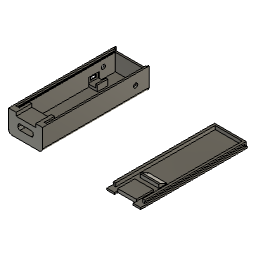
Coco_long_flat_Cover (Autodesk Fusion 360 design; units mm, degrees)
Autodesk Fusion 360 part; units mm, degrees
sketch "Skizze1" plane through (0, 0, 0) normal (0, 0, 1) x (1, 0, 0)
  line L0 (18, 20) -> (38, 20)
  line L1 (38, 20) -> (38, 83)
  line L2 (38, 83) -> (18, 83)
  line L3 (18, 83) -> (18, 20)
  line L4 (19, 23.2) -> (37, 23.2)
  line L5 (37, 23.2) -> (37, 82)
  line L6 (37, 82) -> (19, 82)
  line L7 (19, 82) -> (19, 23.2)
  line L8 (57, 90.4333) -> (57, 15.7858)
  line L9 (77, 82) -> (95, 82)
  line L10 (76, 83) -> (96, 83)
  line L11 (96, 83) -> (96, 20)
  line L12 (77, 23.2) -> (77, 82)
  line L13 (96, 20) -> (76, 20)
  line L14 (95, 82) -> (95, 23.2)
  line L15 (76, 20) -> (76, 83)
  line L16 (78, 81) -> (94, 81)
  line L17 (94, 81) -> (94, 23.2)
  line L18 (78, 23.2) -> (78, 81)
  line L19 (78, 81) -> (78, 83)
  line L20 (94, 81) -> (94, 83)
  line L21 (95, 82) -> (95, 83)
  line L22 (77, 82) -> (77, 83)
  line L23 (95, 23.2) -> (94, 23.2)
  line L24 (77, 23.2) -> (78, 23.2)
  line L25 (-15, -7.8) -> (-15, -6.8)
  line L26 (-15, -6.8) -> (-13, -6.8)
  line L27 (-13, -6.8) -> (-13, -15)
  line L28 (-13, -15) -> (-15, -15)
  line L29 (-15, -15) -> (-15, -14)
  line L30 (-15, -14) -> (-13.6, -14)
  line L31 (-13.6, -14) -> (-13.6, -7.8)
  line L32 (-13.6, -7.8) -> (-15, -7.8)
  dimension "d3" = 63
  dimension "d4" = 20
  dimension "d5" = 1
  dimension "d6" = 1
  dimension "d7" = 19
  dimension "d8" = 59.8
  dimension "d13" = 1
  dimension "d15" = 1
  dimension "d16" = 17
  dimension "d71" = 38
  dimension "d72" = 83
  dimension "d212" = 15
  dimension "d213" = 15
  dimension "d214" = 1
  dimension "d215" = 2
  dimension "d216" = 1.4
  dimension "d217" = 7.2
  dimension "d218" = 8.2
  dimension "d246" = 114
  constraint horizontal L0
  constraint vertical L1
  constraint horizontal L2
  constraint vertical L3
  constraint horizontal L4
  constraint vertical L5
  constraint horizontal L6
  constraint vertical L7
  constraint vertical L8
  constraint symmetric L0.start L8 L11.end
  constraint symmetric L0.end L8 L13.end
  constraint symmetric L1.end L8 L10.start
  constraint symmetric L2.end L8 L10.end
  constraint symmetric L4.start L8 L14.end
  constraint symmetric L4.end L8 L12.start
  constraint symmetric L5.end L8 L9.start
  constraint symmetric L6.end L8 L9.end
  constraint horizontal L16
  constraint vertical L17
  constraint vertical L18
  constraint coincident L10 L19.end
  constraint perpendicular L10 L19
  constraint coincident L10 L20.end
  constraint perpendicular L10 L20
  constraint coincident L10 L21.end
  constraint perpendicular L10 L21
  constraint coincident L10 L22.end
  constraint perpendicular L10 L22
  constraint perpendicular L14 L23
  constraint perpendicular L12 L24
  constraint vertical L25
  constraint perpendicular L25 L26
  constraint perpendicular L26 L27
  constraint perpendicular L27 L28
  constraint perpendicular L28 L29
  constraint perpendicular L27 L30
  constraint perpendicular L30 L31
  constraint perpendicular L25 L32
  constraint collinear L25 L29
  measures "d3" distance of L0 L2
  measures "d4" distance of L1 L3
  measures "d5" distance of L2 L6
  measures "d6" distance of L1 L5
  measures "d7" distance of L1 L7
  measures "d8" distance of L2 L4
  measures "d13" distance of L9 L16
  measures "d15" distance of L14 L17
  measures "d16" distance of L14 L18
  measures "d71" distance of origin L1
  measures "d72" distance of origin L2
  measures "d212" distance of origin L28
  measures "d213" distance of origin L29
  measures "d214" distance of L28 L30
  measures "d215" distance of L27 L29
  measures "d216" distance of L29 L31
  measures "d217" distance of L28 L32
  measures "d218" distance of L26 L28
extrude "Extrusion1" add sketch "Skizze1" along normal blind 13 contours L0 L1 L2 L3 makes body 1
extrude "Extrusion2" add sketch "Skizze1" along normal blind 1 contours L4 L5 L6 L7 bodies 1
extrude "Extrusion3" add sketch "Skizze1" along normal blind 3 separate body contours L9 L10 L19 L22 | L9 L12 L18 L19 L24 | L9 L10 L19 L20 | L9 L10 L20 L21 | L9 L14 L17 L20 L23 makes body 2
extrude "Extrusion4" add sketch "Skizze1" along normal blind 1 contours L9 L10 L19 L22 | L10 L11 L12 L13 L14 L15 L16 L17 L18 L21 L22 L23 L24 | L9 L10 L19 L20 | L9 L16 L19 L20 | L9 L10 L20 L21 bodies 2
fillet "Abrundung1" radius 2 2 edges at (38, 51.5, 0) (18, 51.5, 0) on bodies 1
ref_plane "Arbeitsebene1" through (28, 0, 0) normal (1, 0, 0) x (0, 1, 0)
sketch "Skizze2" plane through (28, 0, 0) normal (1, 0, 0) x (0, 1, 0)
  line L0 (23.2, 12) -> (83, 12)
  line L1 (83, 12) -> (83, 11)
  line L2 (83, 11) -> (23.2, 11)
  line L3 (23.2, 11) -> (23.2, 12)
  dimension "d25" = 11
  dimension "d26" = 59.8
  dimension "d27" = 1
  dimension "d44" = 83
  constraint horizontal L0
  constraint vertical L1
  constraint horizontal L2
  constraint vertical L3
  measures "d25" vertical distance of origin L2.end
  measures "d26" distance of L1 L3
  measures "d27" distance of L0 L2
  measures "d44" distance of origin L1
extrude "Extrusion10" cut sketch "Skizze2" along normal mid plane 19 bodies 1
sketch "Skizze3" plane through (0, 20, 0) normal (0, -1, 0) x (1, 0, 0)
  arc A0 (18, 2) -> (20, 0) centre (20, 2) ccw
  line L0 (20, 0) -> (36, 0)
  arc A1 (36, 0) -> (38, 2) centre (36, 2) ccw
  line L1 (38, 2) -> (38, 13)
  line L2 (38, 13) -> (18, 13)
  line L3 (18, 13) -> (18, 2)
  line L4 (24.69, 4.89) -> (31.31, 4.89)
  line L5 (24.69, 8.11) -> (31.31, 8.11)
  line L6 (28, 12.5188) -> (28, 0.4317)
  arc A2 (23.49, 6.09) -> (24.69, 4.89) centre (24.69, 6.09) ccw
  line L7 (23.49, 6.09) -> (23.49, 6.91)
  arc A3 (24.69, 8.11) -> (23.49, 6.91) centre (24.69, 6.91) ccw
  arc A4 (32.51, 6.91) -> (31.31, 8.11) centre (31.31, 6.91) ccw
  arc A5 (31.31, 4.89) -> (32.51, 6.09) centre (31.31, 6.09) ccw
  line L8 (32.51, 6.91) -> (32.51, 6.09)
  line L9 (22.5, 13) -> (34, 13)
  line L10 (34, 13) -> (34, 11)
  line L11 (34, 11) -> (22.5, 11)
  line L12 (22.5, 11) -> (22.5, 13)
  dimension "d30" = 6.62
  dimension "d31" = 4.89
  dimension "d32" = 6.62
  dimension "d33" = 8.11
  dimension "d34" = 3.31
  dimension "d35" = 3.31
  dimension "d36" = 1.2
  dimension "d37" = 1.2
  dimension "d171" = 2
  dimension "d204" = 6
  dimension "d205" = 11.5
  constraint horizontal L4
  constraint horizontal L5
  constraint tangent L4 A2
  constraint vertical L7
  constraint tangent L7 A3
  constraint tangent L5 A3
  constraint tangent A2 L7
  constraint tangent L5 A4
  constraint tangent L4 A5
  constraint perpendicular L2 L8
  constraint tangent A5 L8
  constraint tangent A4 L8
  constraint horizontal L9
  constraint vertical L10
  constraint horizontal L11
  constraint vertical L12
  constraint coincident L2 L9.start
  measures "d30" distance of L4.start L4.end
  measures "d31" distance of L0 L4
  measures "d32" distance of L5.start L5.end
  measures "d33" distance of L0 L5
  measures "d34" distance of L4.end L6
  measures "d35" distance of L5.end L6
  measures "d36" radius of A3
  measures "d37" radius of A4
  measures "d171" distance of L9 L11
  measures "d204" distance of L6 L10
  measures "d205" distance of L10 L12
extrude "Extrusion6" cut sketch "Skizze3" against normal blind 3.2 contours L2 L9 L10 L11 L12 | L4 L5 L6 A2 L7 A3 | L4 L5 L6 A4 A5 L8 bodies 1
fillet "Abrundung2" [suppressed]
sketch "Skizze7" plane through (0, 83, 0) normal (0, 1, 0) x (-1, 0, 0)
  arc A0 (-20, 0) -> (-18, 2) centre (-20, 2) ccw
  line L0 (-18, 2) -> (-18, 13)
  line L1 (-38, 13) -> (-38, 2)
  arc A1 (-38, 2) -> (-36, 0) centre (-36, 2) ccw
  line L2 (-36, 0) -> (-20, 0)
  line L3 (-37.5, 13) -> (-18.5, 13)
  line L4 (-18.5, 13) -> (-18.5, 12)
  line L5 (-18.5, 12) -> (-37.5, 12)
  line L6 (-37.5, 12) -> (-37.5, 13)
  line L7 (-28, 12.5188) -> (-28, 0.4317)
  circle A2 centre (-31.5, 6) radius 1.25
  line L8 (-18.5, 11) -> (-37.5, 11)
  line L9 (-18.5, 12) -> (-18.5, 11)
  line L10 (-37.5, 11) -> (-37.5, 12)
  line L11 (-37.5, 12) -> (-18.5, 12)
  line L12 (-18, 13) -> (-38, 13)
  dimension "d59" = 19
  dimension "d60" = 9.5
  dimension "d116" = 2.5
  dimension "d117" = 6
  dimension "d206" = 3.5
  dimension "d264" = 13
  dimension "d265" = 1
  constraint horizontal L3
  constraint vertical L4
  constraint horizontal L5
  constraint vertical L6
  measures "d59" distance of L4 L6
  measures "d60" distance of L4 L7
  measures "d116" diameter of A2
  measures "d117" distance of L2 A2.centre
  measures "d206" distance of L7 A2.centre
  measures "d264" distance of origin L3
  measures "d265" distance of L3 L5
extrude "Extrusion11" cut sketch "Skizze7" against normal blind 1 contours L3 L4 L5 L6 L11 L12 bodies 1
sketch "Skizze8" plane through (95, 0, 0) normal (1, 0, 0) x (0, 1, 0)
  line L0 (23.2, 1) -> (83, 1)
  line L1 (83, 1) -> (83, 3)
  line L2 (83, 3) -> (23.2, 3)
  line L3 (23.2, 3) -> (83, 3)
  line L4 (82, 2.1) -> (23.2, 2.1)
  line L5 (23.2, 2.1) -> (23.2, 3)
  line L6 (83, 3) -> (83, 1)
  line L7 (82, 1) -> (82, 2.1)
  line L8 (23.2, 3) -> (23.2, 1)
  dimension "d63" = 0.9
  dimension "d125" = 1
  constraint horizontal L3
  constraint horizontal L4
  constraint vertical L5
  constraint coincident L2.end L3.start
  constraint coincident L0.end L1.start
  constraint coincident L0 L7.start
  constraint coincident L4 L7.end
  constraint perpendicular L4 L7
  constraint coincident L1.end L2.start
  measures "d63" distance of L2.end L4.end
  measures "d125" distance of L6 L7
extrude "Extrusion12" add sketch "Skizze8" along normal blind 0.4 contours L0 L1 L2 L3 L4 L5 L6 L7 L8 bodies 2
sketch "Skizze9" plane through (77, 0, 0) normal (-1, 0, 0) x (0, -1, 0)
  line L0 (-83, 1) -> (-23.2, 1)
  line L1 (-23.2, 3) -> (-83, 3)
  line L2 (-83, 3) -> (-83, 1)
  line L3 (-83, 3) -> (-23.2, 3)
  line L4 (-23.2, 3) -> (-23.2, 2.1)
  line L5 (-23.2, 2.1) -> (-82, 2.1)
  line L6 (-83, 1) -> (-83, 3)
  line L7 (-83, 1) -> (-82, 1)
  line L8 (-82, 2.1) -> (-82, 1)
  line L9 (-23.2, 1) -> (-23.2, 3)
  line L10 (-83, 1) -> (-23.2, 1)
  line L11 (-23.2, 1) -> (-23.2, 3)
  line L12 (-23.2, 3) -> (-83, 3)
  line L13 (-83, 3) -> (-83, 1)
  dimension "d126" = 0.9
  dimension "d127" = 1
  constraint horizontal L3
  constraint vertical L4
  constraint horizontal L5
  constraint vertical L6
  constraint coincident L1.end L2.start
  constraint coincident L0.start L2.end
  constraint coincident L0 L7.end
  constraint coincident L5 L8.start
  constraint perpendicular L0 L8
  constraint coincident L5.end L8
  constraint coincident L1.start L3.end
  measures "d126" distance of L3 L5
  measures "d127" distance of L6 L8
extrude "Extrusion13" add sketch "Skizze9" along normal blind 0.4 contours L0 L1 L2 L3 L4 L5 L6 L7 L8 L9 L10 L11 L12 L13 bodies 2
sketch "Skizze10" plane through (0, 0, 1) normal (0, 0, 1) x (-1, 0, 0)
  line L0 (-76.6, -83) -> (-76, -83)
  line L1 (-76, -20) -> (-96, -20)
  line L2 (-95, -82) -> (-95, -23.2)
  line L3 (-94, -23.2) -> (-94, -82)
  line L4 (-95, -23.2) -> (-94, -23.2)
  line L5 (-95.4, -82) -> (-95, -82)
  line L6 (-95.4, -83) -> (-95.4, -82)
  line L7 (-76, -83) -> (-76, -20)
  line L8 (-96, -20) -> (-96, -83)
  line L9 (-96, -83) -> (-95.4, -83)
  line L10 (-80.5, -32) -> (-91.5, -32)
  line L11 (-80.5, -32) -> (-80.5, -22)
  line L12 (-80.5, -22) -> (-91.5, -22)
  line L13 (-91.5, -22) -> (-91.5, -32)
  line L14 (-80.5, -40.2) -> (-91.5, -40.2)
  line L15 (-91.5, -40.2) -> (-91.5, -35.2)
  line L16 (-91.5, -35.2) -> (-80.5, -35.2)
  line L17 (-80.5, -35.2) -> (-80.5, -40.2)
  line L18 (-77, -23.2) -> (-77, -82)
  line L19 (-78, -82) -> (-78, -23.2)
  line L20 (-78, -23.2) -> (-77, -23.2)
  line L21 (-76.6, -83) -> (-95.4, -83)
  line L22 (-76.6, -82) -> (-76.6, -83)
  line L23 (-77, -82) -> (-76.6, -82)
  dimension "d224" = 4.5
  dimension "d225" = 15.5
  dimension "d226" = 2
  dimension "d227" = 12
  dimension "d249" = 20.2
  dimension "d250" = 15.2
  constraint perpendicular L10 L11
  constraint perpendicular L10 L13
  constraint horizontal L14
  constraint vertical L15
  constraint horizontal L16
  constraint vertical L17
  constraint collinear L11 L17
  constraint collinear L13 L15
  measures "d224" distance of L7 L11
  measures "d225" distance of L7 L13
  measures "d226" distance of L1 L12
  measures "d227" distance of L1 L10
  measures "d249" distance of L1 L14
  measures "d250" distance of L1 L16
extrude "Extrusion30" add sketch "Skizze10" along normal blind 1 contours L10 L11 L12 L13 bodies 2
extrude "Extrusion33" add sketch "Skizze10" along normal blind 2 contours L14 L15 L16 L17 bodies 2
chamfer "Fase2" distance 4 distance2 2 1 edges at (86, 40.2, 3) measured on face at (84.1667, 38.5333, 3) on bodies 2
sketch "Skizze11" plane through (18, 0, 0) normal (-1, 0, 0) x (0, -1, 0)
  line L0 (-83, 2) -> (-20, 2)
  line L1 (-20, 2) -> (-20, 13)
  line L2 (-20, 13) -> (-83, 13)
  line L3 (-83, 13) -> (-83, 2)
  line L4 (-71.2, 3.4) -> (-67.9, 3.4)
  line L5 (-67.9, 3.4) -> (-67.9, 5)
  line L6 (-67.9, 5) -> (-71.2, 5)
  line L7 (-71.2, 5) -> (-71.2, 3.4)
  line L8 (-66.5, 5.95) -> (-66.5, 2.45)
  line L9 (-66.5, 5.95) -> (-72.6, 5.95)
  line L10 (-72.6, 5.95) -> (-72.6, 2.45)
  line L11 (-72.6, 2.45) -> (-66.5, 2.45)
  circle A0 centre (-75, 7) radius 1.25
  dimension "d76" = 3.3
  dimension "d77" = 1.6
  dimension "d78" = 15.1
  dimension "d179" = 3.95
  dimension "d180" = 3.5
  dimension "d181" = 16.5
  dimension "d182" = 6.1
  dimension "d193" = 3
  dimension "d258" = 6
  dimension "d259" = 8
  dimension "d260" = 2.5
  constraint horizontal L4
  constraint vertical L5
  constraint horizontal L6
  constraint vertical L7
  constraint perpendicular L6 L8
  constraint perpendicular L8 L9
  constraint perpendicular L0 L10
  constraint horizontal L11
  measures "d76" distance of L4.start L4.end
  measures "d77" distance of L4.start L6.end
  measures "d78" distance of L3 L5
  measures "d179" distance of L0 L9
  measures "d180" distance of L9 L11
  measures "d181" distance of L3 L8
  measures "d182" distance of L8 L10
  measures "d193" distance of L0 L6
  measures "d258" distance of L2 A0.centre
  measures "d259" distance of L3 A0.centre
  measures "d260" diameter of A0
extrude "Extrusion15" cut sketch "Skizze11" against normal blind 1 contours L4 L5 L6 L7 bodies 1
extrude "Extrusion34" cut sketch "Skizze11" against normal blind 20 contours A0 bodies 1
sketch "Skizze12" plane through (0, 0, 1) normal (0, 0, 1) x (-1, 0, 0)
  line L0 (-19, -82) -> (-19, -23.2)
  line L1 (-19, -23.2) -> (-37, -23.2)
  line L2 (-37, -23.2) -> (-37, -82)
  line L3 (-23, -72.5) -> (-23, -66.4)
  line L4 (-24, -72.5) -> (-24, -66.4)
  line L5 (-24, -66.4) -> (-23, -66.4)
  line L6 (-34, -20) -> (-38, -20)
  line L7 (-18, -20) -> (-22.5, -20)
  line L8 (-24, -72.5) -> (-23, -72.5)
  line L9 (-18, -83) -> (-18, -20)
  line L10 (-23, -72.5) -> (-19, -72.5)
  line L11 (-23, -66.4) -> (-19, -66.4)
  line L12 (-18.5, -83) -> (-18, -83)
  dimension "d177" = 6
  dimension "d178" = 5
  dimension "d253" = 10.5
  dimension "d254" = 16.6
  constraint vertical L3
  constraint perpendicular L4 L5
  constraint vertical L4
  constraint perpendicular L3 L8
  constraint coincident L0 L10.end
  constraint perpendicular L0 L10
  constraint coincident L0 L11.end
  constraint perpendicular L0 L11
  measures "d177" distance of L4 L9
  measures "d178" distance of L3 L9
  measures "d253" distance of L10 L12
  measures "d254" distance of L11 L12
extrude "Extrusion17" add sketch "Skizze12" along normal blind 3.5 contours L3 L4 L5 L8 bodies 1
extrude "Extrusion27" add sketch "Skizze12" along normal blind 1.45 contours L0 L3 L10 L11 bodies 1
sketch "Skizze13" plane through (19, 0, 0) normal (1, 0, 0) x (0, 1, 0)
  line L0 (82, 1) -> (82, 11)
  line L1 (23.2, 11) -> (23.2, 1)
  line L2 (72.5, 1) -> (82, 1)
  line L3 (71.2, 3.4) -> (67.9, 3.4)
  line L4 (67.9, 3.4) -> (67.9, 5)
  line L5 (67.9, 5) -> (71.2, 5)
  line L6 (71.2, 5) -> (71.2, 3.4)
  line L7 (-70.5, 1.05) -> (-64.4, 1.05)
  line L8 (-64.4, 4.55) -> (-64.4, 1.05)
  line L9 (-65.9, 2) -> (-65.9, 3.6)
  line L10 (-69, 2) -> (-65.9, 2)
  line L11 (-64.4, 4.55) -> (-70.5, 4.55)
  line L12 (-70.5, 4.55) -> (-70.5, 1.05)
  line L13 (-69, 3.6) -> (-69, 2)
  line L14 (-65.9, 3.6) -> (-69, 3.6)
  line L15 (66.4, 5.95) -> (66.4, 1)
  line L16 (72.5, 1) -> (72.5, 5.95)
  line L17 (72.5, 5.95) -> (66.4, 5.95)
  line L18 (83, 13) -> (83, 2)
  line L19 (72.6, 2.45) -> (66.5, 2.45)
  line L20 (72.5, 2.45) -> (72.5, 1)
  line L21 (66.4, 1) -> (66.4, 2.45)
  line L22 (66.4, 2.45) -> (72.5, 2.45)
  line L23 (23.2, 1) -> (66.4, 1)
  line L24 (82, 11) -> (23.2, 11)
  circle A0 centre (75, 7) radius 1.25
  point P0 (-83, 2)
  dimension "d183" = 3.1
  dimension "d184" = 1.6
  dimension "d185" = 3.5
  dimension "d186" = 6.1
  dimension "d187" = 6.1
  dimension "d188" = 16.6
  dimension "d189" = 3.5
  constraint horizontal L10
  constraint vertical L9
  constraint horizontal L14
  constraint vertical L13
  constraint perpendicular L8 L14
  constraint perpendicular L8 L11
  constraint horizontal L7
  constraint coincident L2 L15.end
  constraint perpendicular L2 L15
  constraint coincident L2 L16.start
  constraint perpendicular L2 L16
  constraint perpendicular L15 L17
  measures "d183" distance of L10.start L9.start
  measures "d184" distance of L10.start L13.start
  measures "d185" distance of L7 L11
  measures "d186" distance of L8 L12
  measures "d187" distance of L15 L16
  measures "d188" distance of L15 L18
  measures "d189" distance of L17 L19
extrude "Extrusion26" cut sketch "Skizze13" against normal blind 0.5 contours L15 L16 L17 L19 L22 bodies 1
sketch "Skizze14" plane through (0, 20, 0) normal (0, -1, 0) x (1, 0, 0)
  line L0 (76, 0) -> (96, 0)
  line L1 (96, 1) -> (76, 1)
  line L2 (80.5, 1) -> (91.5, 1)
  line L3 (91.5, 1) -> (91.5, 0)
  line L4 (91.5, 0) -> (80.5, 0)
  line L5 (80.5, 0) -> (80.5, 1)
  line L6 (96, 0) -> (96, 1)
  line L7 (76, 1) -> (76, 0)
  dimension "d105" = 15.5
  dimension "d106" = 11
  dimension "d107" = 1
  constraint horizontal L2
  constraint vertical L3
  constraint horizontal L4
  constraint vertical L5
  constraint coincident L1 L2.start
  measures "d105" distance of L1.end L3
  measures "d106" distance of L3 L5
  measures "d107" distance of L1 L4
extrude "Extrusion20" cut sketch "Skizze14" against normal blind 2 contours L0 L1 L2 L3 L4 L5 bodies 2
ref_plane "Arbeitsebene2" through (0, 0, 6) normal (0, 0, 1) x (1, 0, 0)
sketch "Skizze15" plane through (0, 0, 6) normal (0, 0, 1) x (1, 0, 0)
  line L0 (24, 83) -> (24, 86)
  arc A0 (27, 89) -> (24, 86) centre (27, 86) ccw
  arc A1 (34, 86) -> (31, 89) centre (31, 86) ccw
  line L1 (27, 89) -> (31, 89)
  line L2 (34, 86) -> (34, 83)
  line L3 (18, 83) -> (18, 20)
  line L4 (18.5, 83) -> (18, 83)
  dimension "d112" = 16
  dimension "d113" = 10
  dimension "d114" = 3
  dimension "d115" = 3
  dimension "d255" = 3
  constraint vertical L0
  constraint tangent L0 A0
  constraint tangent A0 L1
  constraint perpendicular L1 L2
  constraint tangent A1 L1
  constraint tangent A1 L2
  constraint vertical L2
  measures "d112" distance of L2 L3
  measures "d113" distance of L0 L2
  measures "d114" radius of A0
  measures "d115" radius of A1
  measures "d255" distance of A0.centre L4
sweep "Sweeping1" [suppressed]
fillet "Abrundung5" [suppressed]
sketch "Skizze16" plane through (0, 0, 0) normal (0, 0, -1) x (1, 0, 0)
  line L0 (20, -20) -> (20, -83)
  line L1 (20, -83) -> (36, -83)
  line L2 (36, -83) -> (36, -20)
  line L3 (36, -20) -> (20, -20)
  circle A0 centre (28, -28) radius 7
  circle A1 centre (28, -28) radius 6
  line L4 (38, -83) -> (38, -20)
  circle A2 centre (28, -28) radius 3
  circle A3 centre (28, -28) radius 1.5
  line L5 (22.9049, -23.2) -> (33.0951, -23.2)
  dimension "d128" = 14
  dimension "d129" = 8
  dimension "d130" = 10
  dimension "d131" = 1
  dimension "d132" = 6
  dimension "d133" = 3
  dimension "d263" = 3.2
  constraint concentric A0 A1
  constraint concentric A0 A2
  constraint concentric A1 A3
  constraint coincident A0 L5.start
  constraint coincident A0 L5.end
  constraint horizontal L5
  measures "d128" diameter of A0
  measures "d129" distance of L3 A0.centre
  measures "d130" distance of A0.centre L4
  measures "d131" distance of A0 A1
  measures "d132" diameter of A2
  measures "d133" diameter of A3
  measures "d263" distance of L3 L5
extrude "Extrusion32" cut sketch "Skizze16" against normal blind 1 contours A0 A1 L5 | A2 | A3 picked at (23.4498, -32.8545) bodies 1
extrude "Extrusion22" add sketch "Skizze16" against normal blind 1 separate body contours A0 A1 L5 | A2 | A3 picked at (23.4498, -32.8545) makes body 3 at (27.9253, 27.1355, 0) makes body 4 at (23.8756, 33.6559, 0.6667)
sketch "Skizze17" plane through (0, 23.2, 0) normal (0, 1, 0) x (-1, 0, 0)
  line L0 (-37, 13) -> (-37, 12)
  line L1 (-37, 1) -> (-33.0951, 1)
  line L2 (-19, 1) -> (-19, 11)
  line L3 (-19, 9.11) -> (-37, 9.11)
  line L4 (-37, 9.11) -> (-37, 10.11)
  line L5 (-37, 10.11) -> (-19, 10.11)
  line L6 (-19, 10.11) -> (-19, 9.11)
  line L7 (-23.49, 6.91) -> (-23.49, 6.09)
  arc A0 (-24.69, 4.89) -> (-23.49, 6.09) centre (-24.69, 6.09) ccw
  line L8 (-24.69, 4.89) -> (-31.31, 4.89)
  arc A1 (-32.51, 6.09) -> (-31.31, 4.89) centre (-31.31, 6.09) ccw
  line L9 (-32.51, 6.09) -> (-32.51, 6.91)
  arc A2 (-31.31, 8.11) -> (-32.51, 6.91) centre (-31.31, 6.91) ccw
  line L10 (-31.31, 8.11) -> (-24.69, 8.11)
  arc A3 (-23.49, 6.91) -> (-24.69, 8.11) centre (-24.69, 6.91) ccw
  line L11 (-21.1, 13) -> (-21.1, 12)
  line L12 (-35.9, 12) -> (-35.9, 13)
  line L13 (-37, 12) -> (-37, 13)
  line L14 (-19, 12) -> (-19, 13)
  line L15 (-22.5, 13) -> (-22.5, 11)
  line L16 (-34, 11) -> (-34, 13)
  line L17 (-34, 13) -> (-37, 13)
  line L18 (-38, 2) -> (-38, 13)
  line L19 (-34, 11) -> (-22.5, 11)
  line L20 (-35, 10.11) -> (-35, 12)
  line L21 (-35.9, 12) -> (-35, 12)
  line L22 (-21.5, 12) -> (-21.1, 12)
  line L23 (-21.1, 13) -> (-22.5, 13)
  line L24 (-21.5, 12) -> (-21.5, 10.11)
  line L25 (-35.9, 13) -> (-34, 13)
  line L26 (-34, 11) -> (-22.5, 11)
  line L27 (-19, 13) -> (-22.5, 13)
  line L28 (-37, 12) -> (-37.5, 12)
  line L29 (-37.5, 11) -> (-37, 11)
  line L30 (-37, 11) -> (-37, 1)
  line L31 (-19, 11) -> (-18.5, 11)
  line L32 (-19, 12) -> (-19, 13)
  line L33 (-37.5, 12) -> (-37.5, 11)
  line L34 (-18.5, 11) -> (-18.5, 12)
  line L35 (-18.5, 12) -> (-19, 12)
  line L36 (-18.5, 12) -> (-19, 12)
  line L37 (-37, 12) -> (-37.5, 12)
  line L38 (-33.0951, 1) -> (-33.0951, 0)
  line L39 (-33.0951, 0) -> (-31.6, 0)
  line L40 (-31.6, 0) -> (-31.6, 1)
  line L41 (-31.6, 1) -> (-24.4, 1)
  line L42 (-24.4, 1) -> (-24.4, 0)
  line L43 (-24.4, 0) -> (-22.9049, 0)
  line L44 (-22.9049, 0) -> (-22.9049, 1)
  line L45 (-22.9049, 1) -> (-19, 1)
  line L46 (-22.5, 13) -> (-19, 13)
  line L47 (-37, 13) -> (-34, 13)
  dimension "d165" = 1
  dimension "d166" = 2
  dimension "d174" = 2.1
  dimension "d175" = 16.9
  dimension "d210" = 1
  dimension "d211" = 1
  dimension "d266" = 1
  constraint horizontal L3
  constraint vertical L4
  constraint horizontal L5
  constraint vertical L6
  constraint coincident L0 L4.end
  constraint coincident L2 L3.start
  constraint vertical L11
  constraint vertical L12
  constraint coincident L16.start L19.start
  constraint coincident L15.end L19.end
  constraint perpendicular L20 L21
  constraint vertical L20
  constraint coincident L5 L20.start
  constraint perpendicular L11 L22
  constraint coincident L15.start L23.end
  constraint coincident L5 L24.end
  constraint perpendicular L5 L24
  constraint coincident L16.end L17.start
  constraint collinear L21 L22
  measures "d165" distance of L3 L10
  measures "d166" distance of L5 L10
  measures "d174" distance of L12 L18
  measures "d175" distance of L11 L18
  measures "d210" distance of L15 L24
  measures "d211" distance of L16 L20
  measures "d266" distance of L21 L25
extrude "Extrusion25" add sketch "Skizze17" along normal blind 6 contours L5 L11 L12 L15 L16 L17 L19 L20 L21 L22 L23 L24 L25 L26 L27 L46 L47 bodies 1
extrude "Extrusion28" add sketch "Skizze1" along normal blind 4 separate body contours L25 L26 L27 L28 L29 L30 L31 L32 makes body 5
sketch "Skizze18" plane through (-13.6, 0, 0) normal (-1, 0, 0) x (0, -1, 0)
  line L0 (7.8, 0) -> (14, 0)
  line L1 (14, 0) -> (14, 4)
  line L2 (14, 4) -> (7.8, 4)
  line L3 (7.8, 4) -> (7.8, 0)
  line L4 (7.8, 0) -> (14, 0)
  line L5 (14, 0) -> (14, 1.5)
  line L6 (14, 1.5) -> (7.8, 1.5)
  line L7 (7.8, 1.5) -> (7.8, 0)
  dimension "d221" = 1.5
  constraint horizontal L4
  constraint vertical L5
  constraint horizontal L6
  constraint vertical L7
  constraint coincident L1 L5.end
  constraint coincident L0.start L3.end
  measures "d221" distance of L4 L6
extrude "Extrusion29" cut sketch "Skizze18" against normal blind 0.6 contours L0 L1 L3 L4 L5 L6 L7 bodies 5
sketch "Skizze19" plane through (0, 0, 6) normal (0, 0, 1) x (1, 0, 0)
  circle A0 centre (29, 90) radius 10
  line L0 (18, 83) -> (18, 20)
  line L1 (14, 105) -> (44, 105)
  line L2 (44, 105) -> (44, 83)
  line L3 (14, 83) -> (14, 105)
  line L4 (18.5, 83) -> (18, 83)
  line L5 (44, 83) -> (14, 83)
  dimension "d231" = 20
  dimension "d233" = 11
  dimension "d234" = 15
  dimension "d235" = 30
  dimension "d236" = 15
  dimension "d256" = 7
  dimension "d257" = 7
  constraint horizontal L1
  constraint vertical L2
  constraint vertical L3
  constraint perpendicular L3 L5
  measures "d231" diameter of A0
  measures "d233" distance of A0.centre L0
  measures "d234" distance of A0.centre L2
  measures "d235" distance of L2 L3
  measures "d236" distance of A0.centre L1
  measures "d256" distance of A0.centre L4
  measures "d257" distance of A0.centre L5
hidden bodies 3 4 5
equation "d3 = Länge + Wandstärke"
equation "d4 = Breite + 2 * Wandstärke"
equation "d5 = Wandstärke"
equation "d6 = Wandstärke"
equation "d7 = Breite + Wandstärke"
equation "d8 = d3 - 3.2 mm"
equation "d9 = Höhe_Gehäuse"
equation "d11 = Wandstärke"
equation "d16 = Breite - 1 mm"
equation "d17 = Höhe_Deckel + 2 mm"
equation "d19 = Höhe_Deckel"
equation "d23 = Breite + 20 mm - Breite / 2 - Wandstärke"
equation "d25 = Höhe_Gehäuse - 2 mm"
equation "d26 = Länge + Wandstärke - 3.2 mm"
equation "d30 = d34 * 2"
equation "d32 = d30"
equation "d35 = d34"
equation "d44 = Länge + Wandstärke + 20 mm"
equation "d56 = Höhe_Deckel"
equation "d57 = Breite / 2 + 0.5 mm"
equation "d59 = Breite + 1 mm"
equation "d60 = Breite / 2 + 0.5 mm"
equation "d71 = Breite + 20 mm"
equation "d72 = Länge + 21 mm"
equation "d79 = -Wandstärke"
equation "d105 = Breite / 4 + 11 mm"
equation "d107 = Höhe_Deckel"
equation "d130 = Breite / 2 + Wandstärke"
equation "d175 = Breite - 1.1 mm"
equation "d178 = d177 - 1 mm"
equation "d179 = d193 - d77 / 2 + d180 / 2"
equation "d181 = d78 + d182 / 2 - d76 / 2"
equation "Länge = 62 mm"
equation "Breite = 18 mm"
equation "Wandstärke = 1 mm"
equation "Höhe_Gehäuse = 13 mm"
equation "Höhe_Deckel = 1 mm"
equation "d216 = d215 - 0.6 mm"
equation "d217 = d218 - 1 mm"
equation "d224 = Breite / 4"
equation "d225 = d224 + 11 mm"
equation "d234 = d231 / 2 + 5 mm"
equation "d235 = d234 * 2"
equation "d236 = d231 / 2 + 5 mm"
equation "d246 = d71 * 3"
equation "d249 = d250 + 5 mm"
equation "d253 = Wandstärke + 9.5 mm"
equation "d254 = Wandstärke + 15.6 mm"
equation "d258 = Höhe_Gehäuse / 2 - 0.5 mm"
equation "d261 = -Breite - 2 * Wandstärke"
equation "d264 = Höhe_Gehäuse"
named bodies: "Gehäuse", "Deckel"
